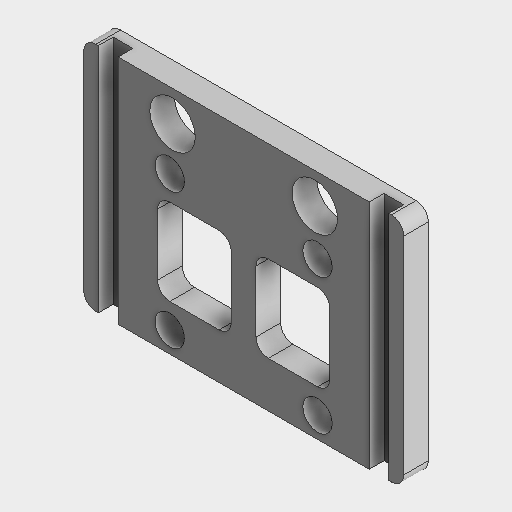
# Autodesk Inventor part: z plate bracket
Saved by Autodesk Inventor 2019 (Build 230136000, 136)
## iProperties
Created: 2017-10-06
Part Number: z plate bracket
Material: Generic
Document SubType Name: Modeling
Designer: MISAKA
Density: 1 g/cm^3
Appearance: Default
Author: MISAKA
Autodesk Inventor part; units mm, degrees
ref_plane "YZ Plane" through (0, 0, 0) normal (1, 0, 0) x (0, 1, 0)
ref_plane "XZ Plane" through (0, 0, 0) normal (0, 1, 0) x (-1, 0, 0)
ref_plane "XY Plane" through (0, 0, 0) normal (0, 0, 1) x (1, 0, 0)
sketch "Sketch1" plane through (0, 0, 0) normal (0, 0, 1) x (1, 0, 0)
  line L0 (-91, 0) -> (91, 0) construction
  line L1 (0, -94.2771) -> (0, 159.6624) construction
  circle A0 centre (-30, 27.5) radius 6
  circle A1 centre (30, 27.5) radius 6
  line L2 (-30, 27.5) -> (30, 27.5) construction
  line L3 (30, 27.5) -> (30, -27.5) construction
  line L4 (30, -27.5) -> (-30, -27.5) construction
  line L5 (-30, -27.5) -> (-30, 27.5) construction
  circle A2 centre (-30, -27.5) radius 6
  circle A3 centre (30, -27.5) radius 6
  line L6 (-30, 17.5) -> (-5, 17.5)
  line L7 (-5, 17.5) -> (-5, -17.5)
  line L8 (-5, -17.5) -> (-30, -17.5)
  circle A4 centre (-30, 0) radius 5
  circle A5 centre (-13, 7.5) radius 5.5
  circle A6 centre (-13, -7.5) radius 5.5
  line L9 (-45, 36) -> (45, 36)
  line L10 (45, 36) -> (45, -36)
  line L11 (45, -36) -> (-45, -36)
  line L12 (-45, -36) -> (-45, 36)
  circle A7 centre (-28.9, 45.5) radius 9.25
  circle A8 centre (28.9, 45.5) radius 9.25
  circle A9 centre (-28.9, -45.5) radius 9.25 construction
  circle A10 centre (28.9, -45.5) radius 9.25 construction
  line L13 (-30, 17.5) -> (-35, 17.5)
  line L14 (-35, 17.5) -> (-35, -17.5)
  line L15 (-35, -17.5) -> (-30, -17.5)
  line L16 (-45, 58) -> (45, 58)
  line L17 (45, 58) -> (45, 36)
  line L18 (45, 36) -> (-45, 36)
  line L19 (-45, 36) -> (-45, 58)
  line L20 (-45, -36) -> (45, -36)
  line L21 (45, -36) -> (45, -58) construction
  line L22 (45, -58) -> (-45, -58) construction
  line L23 (-45, -58) -> (-45, -36) construction
  line L24 (-45, -36) -> (-65, -36)
  line L25 (-65, -36) -> (-65, 58)
  line L26 (-65, 58) -> (-45, 58)
  line L27 (-45, 58) -> (-45, -36)
  line L28 (65, -36) -> (45, -36)
  line L29 (45, -36) -> (45, 58)
  line L30 (45, 58) -> (65, 58)
  line L31 (65, 58) -> (65, -36)
  line L32 (-51, -36) -> (-59, -36)
  line L33 (-59, -36) -> (-59, 58)
  line L34 (-59, 58) -> (-51, 58)
  line L35 (-51, 58) -> (-51, -36)
  line L36 (51, -36) -> (59, -36)
  line L37 (59, -36) -> (59, 58)
  line L38 (59, 58) -> (51, 58)
  line L39 (51, 58) -> (51, -36)
  point P0 (0, 0)
  point P1 (-55, 58)
  point P2 (55, 58)
  dimension "d2" = 12
  dimension "d3" = 60
  dimension "d4" = 55
  dimension "d5" = 10
  dimension "d6" = 25
  dimension "d7" = 10
  dimension "d8" = 17
  dimension "d9" = 11
  dimension "d10" = 15
  dimension "d12" = 18
  dimension "d13" = 18.5
  dimension "d14" = 90
  dimension "d15" = 72
  dimension "d18" = 30
  dimension "d25" = 10
  dimension "d26" = 10
  dimension "d28" = 22
  dimension "d35" = 57.8
  dimension "d36" = 20
  dimension "d37" = 8
  constraints: 76 end point, 16 parallel, 12 perpendicular, 11 centre point, 10 horizontal, 6 point on line, 5 midpoint, 5 symmetric about line, 3 collinear, 13 other
  measures "d2" diameter of A0
  measures "d3" distance of L2.start L2.end
  measures "d4" distance of L2.end L3.end
  measures "d5" distance between parallel lines of L6 L2
  measures "d6" distance of L6.start L6.end
  measures "d7" diameter of A4
  measures "d8" horizontal distance of A5.centre A4.centre
  measures "d9" diameter of A5
  measures "d10" distance of A6.centre A5.centre
  measures "d12" vertical distance of L2.start A7.centre
  measures "d13" diameter of A7
  measures "d14" distance of L9.start L9.end
  measures "d15" distance of L9.end L10.end
  measures "d18" distance between parallel lines of L7 L14
  measures "d25" distance between parallel lines of L12 L14
  measures "d26" diameter of L7 L1
  measures "d28" distance of L9.start L16.start
  measures "d35" distance of A7.centre A8.centre
  measures "d36" distance between parallel lines of L25 L12
  measures "d37" distance between parallel lines of L33 L35
extrude "Extrusion1" add sketch "Sketch1" against normal blind 10 contours A0 | A1 | A2 | A3 | A4 | L6 L7 L8 L15 L14 L13 | A5 | A6 | L19 L16 L17 L9 | L9 L10 L11 L12 | L12 L24 L35 L26 L19 | L17 L30 L39 L28 L10 | L24 L33 L26 L35 | L39 L30 L37 L28 | L24 L25 L26 L33 | L37 L30 L31 L28
extrude "Extrusion3" cut sketch "Sketch1" against normal through all contours A0 | A1 | A2 | A3
sketch "Sketch2" plane through (0, 0, 0) normal (0, 0, 1) x (1, 0, 0)
  line L0 (-78.9863, 0) -> (78.9863, 0) projected
  line L1 (0, -92.6147) -> (0, 159.3853) projected
  line L2 (-56.4188, 123.3853) -> (56.4188, 123.3853)
  line L3 (56.4188, 123.3853) -> (56.4188, 99.2325)
  line L4 (56.4188, -56.6147) -> (-56.4188, -56.6147)
  line L5 (-56.4188, -56.6147) -> (-56.4188, 99.2325)
  line L6 (-56.4188, 99.2325) -> (56.4188, 99.2325)
  line L7 (56.4188, 99.2325) -> (56.4188, -56.6147)
  line L8 (-56.4188, 99.2325) -> (-56.4188, 123.3853)
  point P0 (0, 0)
  dimension "d27" = 180
  constraints: 14 end point, 5 parallel, 2 horizontal, 2 perpendicular, 1 other
  measures "d27" distance of L2.end L4.start
extrude "Extrusion4" cut sketch "Sketch1" against normal through all contours A4 | A5 | A6
extrude "Extrusion5" cut sketch "Sketch1" against normal through all contours L6 L7 L8 L15 L14 L13
mirror "Mirror2" about plane through (0, 0, 0) normal (1, 0, 0) of "Extrusion4", "Extrusion5"
fillet "Fillet4" radius 5 8 edges at (-35, 17.5, -5) (-5, 17.5, -5) (-35, -17.5, -5) (-5, -17.5, -5) (5, -17.5, -5) (5, 17.5, -5) (35, 17.5, -5) (35, -17.5, -5)
extrude "Extrusion6" cut sketch "Sketch1" against normal blind 6 contours L24 L33 L26 L35 | L39 L30 L37 L28
fillet "Fillet5" radius 5 4 edges at (-65, -36, -5) (65, -36, -5) (65, 58, -5) (-65, 58, -5)
body "Solid1"
